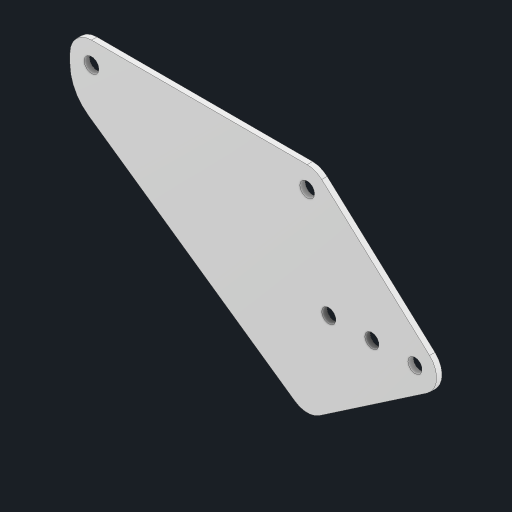
# Autodesk Inventor part: sled
Saved by Autodesk Inventor 2024 (Build 280153000, 153)
## iProperties
Created: 2024-03-11
Part Number: sled
Material: Acetal Resin, White
Document SubType Name: Modeling
Designer: Averey Ku
Density: 1.425 g/cm^3
Appearance: Smooth - White
Author: Averey Ku
Autodesk Inventor part; units mm, degrees
ref_plane "YZ Plane" through (0, 0, 0) normal (1, 0, 0) x (0, 1, 0)
ref_plane "XZ Plane" through (0, 0, 0) normal (0, 1, 0) x (-1, 0, 0)
ref_plane "XY Plane" through (0, 0, 0) normal (0, 0, 1) x (1, 0, 0)
sketch "main" plane through (0, 0, 0) normal (0, 0, 1) x (1, 0, 0)
  circle A0 centre (-16.6212, -19.5437) radius 2.1844
  arc A1 (-20.9032, -24.2328) -> (-16.6212, -25.8937) centre (-16.6212, -19.5437) ccw
  circle A2 centre (-22.9712, 9.4504) radius 2.0955
  arc A3 (-13.0318, 36.2391) -> (-20.24, 36.2816) centre (-16.6667, 31.0324) ccw
  line L0 (-20.9032, -24.2328) -> (-52.6534, 4.7613)
  circle A4 centre (-35.6713, 9.4504) radius 2.0955
  circle A5 centre (-48.3714, 9.4504) radius 2.0955
  arc A6 (-51.9447, 14.6996) -> (-52.6534, 4.7613) centre (-48.3714, 9.4504) ccw
  line L1 (-20.24, 36.2816) -> (-51.9447, 14.6996)
  circle A7 centre (46.8788, -19.5437) radius 2.1844
  arc A8 (46.8788, -25.8937) -> (53.2288, -19.5437) centre (46.8788, -19.5437) ccw
  line L2 (47.7986, -6.2278) -> (-13.0318, 36.2391)
  line L3 (46.8788, -25.8937) -> (-16.6212, -25.8937)
  arc A9 (53.2288, -16.6412) -> (47.7986, -6.2278) centre (40.5288, -16.6412) ccw
  line L4 (53.2288, -19.5437) -> (53.2288, -16.6412)
  point P0 (0.102, -2.5446)
  point P1 (53.2288, -10.0187)
  dimension "d0" = 12.7
  dimension "d1" = 9.525
  dimension "d2" = 12.7
  dimension "d3" = 12.7
  dimension "d4" = 6.35
  dimension "d5" = 4.191
  dimension "d6" = 4.191
  dimension "d7" = 4.191
  measures "d0" diameter of A8
  measures "d1" distance of L4.start point (53.229, -10.019)
  measures "d2" radius of A9
  measures "d3" diameter of A6
  measures "d4" radius of A3
  measures "d5" diameter of A2
  measures "d6" diameter of A4
  measures "d7" diameter of A5
sketch "Sketch1" plane through (0, 0, 0) normal (0, 0, 1) x (1, 0, 0)
  circle A0 centre (63.5, 0) radius 2.1844
  arc A1 (67.782, 4.689) -> (63.5, 6.35) centre (63.5, 0) ccw
  circle A2 centre (69.85, -28.9941) radius 2.0955
  arc A3 (59.9106, -55.7828) -> (67.1187, -55.8253) centre (63.5455, -50.5761) ccw
  line L0 (67.782, 4.689) -> (99.5322, -24.3051)
  circle A4 centre (82.55, -28.9941) radius 2.0955
  circle A5 centre (95.2502, -28.9941) radius 2.0955
  arc A6 (98.8235, -34.2433) -> (99.5322, -24.3051) centre (95.2502, -28.9941) ccw
  line L1 (67.1187, -55.8253) -> (98.8235, -34.2433)
  circle A7 centre (0, 0) radius 2.1844
  arc A8 (0, 6.35) -> (-6.35, 0) centre (0, 0) ccw
  line L2 (-0.9198, -13.3159) -> (59.9106, -55.7828)
  line L3 (0, 6.35) -> (63.5, 6.35)
  arc A9 (-6.35, -2.9025) -> (-0.9198, -13.3159) centre (6.35, -2.9025) ccw
  line L4 (-6.35, 0) -> (-6.35, -2.9025)
  point P0 (0, 0)
  constraints: 1 other
extrude "Extrusion1" add sketch "Sketch1" along normal blind 1.5875
body "Solid1"
